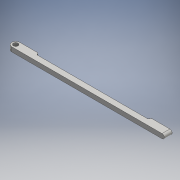
# Autodesk Inventor part: Potentiometer Pushrod
Saved by Autodesk Inventor 2016 (Build 200138000, 138)
## iProperties
Created: 2017-04-03
Part Number: Potentiometer Pushrod
Material: Generic
Document SubType Name: Modeling
Designer: BenjaPad
Density: 1 g/cm^3
Appearance: Default
Author: BenjaPad
Autodesk Inventor part; units mm, degrees
ref_plane "YZ Plane" through (0, 0, 0) normal (1, 0, 0) x (0, 1, 0)
ref_plane "XZ Plane" through (0, 0, 0) normal (0, 1, 0) x (-1, 0, 0)
ref_plane "XY Plane" through (0, 0, 0) normal (0, 0, 1) x (1, 0, 0)
sketch "Sketch1" plane through (0, 0, 0) normal (0, 0, 1) x (1, 0, 0)
  circle A0 centre (0, 0) radius 2.1
  arc A1 (0, 3.5) -> (0, -3.5) centre (0, 0) ccw
  line L0 (0, 3.5) -> (136, 3.5)
  line L1 (136, 3.5) -> (136, -3.5)
  line L2 (136, -3.5) -> (0, -3.5)
  dimension "d0" = 4.2
  dimension "d1" = 7
  dimension "d2" = 136
  constraints: 6 end point, 2 centre point, 2 coincident, 2 point on circle, 1 horizontal, 1 perpendicular, 1 tangent
  measures "d0" diameter of A0
  measures "d1" diameter of A1
  measures "d2" distance from line of point (0, 0) L1
extrude "Extrusion1" add sketch "Sketch1" along normal blind 4
sketch "Sketch2" plane through (0, 3.5, 0) normal (0, 1, 0) x (1, 0, 0)
  line L0 (136, 0) -> (0, 0) projected
  line L1 (0, 0) -> (0, -4) projected
  line L2 (136, -4) -> (0, -4) projected
  line L3 (136, 0) -> (136, -4) projected
  line L4 (134, -2.75) -> (126, -2.75)
  line L5 (126, -2.75) -> (126, -1.25)
  line L6 (126, -1.25) -> (134, -1.25)
  line L7 (134, -1.25) -> (134, -2.75)
  line L8 (134, -2.75) -> (126, -1.25) construction
  line L9 (126, -2.75) -> (134, -1.25) construction
  point P0 (130, -2)
  dimension "d5" = 8
  dimension "d6" = 1.5
  dimension "d7" = 130
  constraints: 12 end point, 2 midpoint, 2 parallel, 1 horizontal, 1 perpendicular
  measures "d5" distance of L5.end L6.end
  measures "d6" distance of L4.end L5.end
  measures "d7" horizontal distance of point (0, 0) point (130, -2)
extrude "Extrusion2" cut sketch "Sketch2" against normal blind 6 contours L4 L5 L6 L7
fillet "Fillet1" radius 2 2 edges at (136, 0, 4) (136, 0, 0)
sketch "Sketch3" plane through (0, 0, 4) normal (0, 0, 1) x (1, 0, 0)
  line L0 (134, 3.5) -> (134, -3.5) projected
  line L1 (134, 3.5) -> (0, 3.5) projected
  arc A0 (0, 3.5) -> (0, -3.5) centre (0, 0) ccw projected
  line L2 (0, -3.5) -> (134, -3.5) projected
  circle A1 centre (0, 0) radius 2.1 projected
  line L3 (126, 3.5) -> (126, -2.5) projected
  line L4 (17, 5.5) -> (117, 5.5)
  line L5 (117, 5.5) -> (117, 1.5)
  line L6 (117, 1.5) -> (17, 1.5)
  line L7 (17, 1.5) -> (17, 5.5)
  line L8 (134, 3.5) -> (0, 3.5) projected
  line L9 (17, 5.5) -> (117, 1.5) construction
  line L10 (117, 5.5) -> (17, 1.5) construction
  point P0 (67, 3.5)
  dimension "d11" = 100
  dimension "d12" = 4
  constraints: 12 end point, 3 midpoint, 2 parallel, 1 horizontal, 1 perpendicular
  measures "d11" distance of L5.end L6.end
  measures "d12" distance of L4.end L5.end
extrude "Extrusion3" cut sketch "Sketch3" against normal blind 6 contours L5 L6 L7 L1 | L1 L7 L4 L5
fillet "Fillet2" radius 1 4 edges at (17, 1.5, 2) (17, 3.5, 2) (117, 3.5, 2) (117, 1.5, 2)
body "Solid1"
